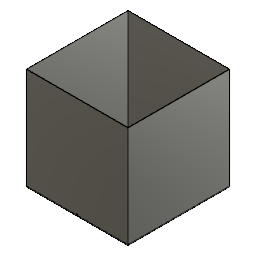
cubical_box_v1 (Autodesk Fusion 360 design; units mm, degrees)
Autodesk Fusion 360 part; units mm, degrees
sketch "Sketch1" plane through (0, 0, 0) normal (0, 1, 0) x (1, 0, 0)
  line L0 (300, -300) -> (-300, -300)
  line L1 (-300, -300) -> (-300, 300)
  line L2 (-300, 300) -> (300, 300)
  line L3 (300, 300) -> (300, -300)
  line L4 (300, -300) -> (-300, 300) construction
  line L5 (-300, -300) -> (300, 300) construction
  dimension "d1" = 600
  dimension "d2" = 600
  constraint perpendicular L0 L1
  constraint parallel L0 L2
  constraint parallel L1 L3
  constraint horizontal L0
  constraint coincident L4 origin
  constraint coincident L5 origin
  measures "d1" distance of L0.end L1.end
  measures "d2" distance of L1.end L2.end
extrude "Extrude1" add sketch "Sketch1" along normal blind 600 in component "Component"
sketch "Sketch2" plane through (0, 600, 0) normal (0, 1, 0) x (-1, 0, 0)
  line L0 (-300, -300) -> (300, -300)
  line L1 (300, -300) -> (300, 300)
  line L2 (300, 300) -> (-300, 300)
  line L3 (-300, 300) -> (-300, -300)
  line L4 (-297.5, 297.5) -> (297.5, 297.5)
  line L5 (297.5, 297.5) -> (297.5, -297.5)
  line L6 (297.5, -297.5) -> (-297.5, -297.5)
  line L7 (-297.5, -297.5) -> (-297.5, 297.5)
  line L8 (-297.5, 297.5) -> (297.5, -297.5) construction
  line L9 (297.5, 297.5) -> (-297.5, -297.5) construction
  dimension "d5" = 595
  dimension "d6" = 595
  constraint perpendicular L4 L5
  constraint parallel L4 L6
  constraint parallel L5 L7
  constraint horizontal L4
  constraint coincident L8 origin
  constraint coincident L9 origin
  measures "d5" distance of L5.end L6.end
  measures "d6" distance of L4.start L6.end
extrude "Extrude2" cut sketch "Sketch2" against normal blind 595 contours L4 L5 L6 L7 in component "Component"
sketch "Sketch3" plane through (0, 0, 300) normal (0, 0, 1) x (1, 0, 0)
  line L0 (-300, 0) -> (300, 0)
  line L1 (300, 0) -> (300, 600)
  line L2 (300, 600) -> (-300, 600)
  line L3 (-300, 600) -> (-300, 0)
  circle A0 centre (0, 9) radius 4
  point P0 (0, 5)
  point P1 (0, 9)
  dimension "d9" = 5
  dimension "d10" = 4
  dimension "d11" = 8
  constraint coincident P1 A0.centre
  measures "d9" distance of origin P0
  measures "d10" distance of P0 P1
  measures "d11" diameter of A0
extrude "Extrude3" cut sketch "Sketch3" against normal blind 30 contours A0 in component "Component"
component "Component" placed x (1, 0, 0) y (0, 1, 0) z (0, 0, 1) at (0, 0, 0)
